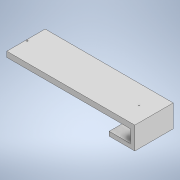
# Autodesk Inventor part: kamera_feste
Saved by Autodesk Inventor 2022 (Build 260153000, 153)
## iProperties
Created: 2022-02-27
Part Number: kamera_feste
Material: Generic
Document SubType Name: Modeling
Designer: eivin
Density: 1 g/cm^3
Appearance: Default
Author: eivin
Autodesk Inventor part; units mm, degrees
ref_plane "YZ Plane" through (0, 0, 0) normal (1, 0, 0) x (0, 1, 0)
ref_plane "XZ Plane" through (0, 0, 0) normal (0, 1, 0) x (-1, 0, 0)
ref_plane "XY Plane" through (0, 0, 0) normal (0, 0, 1) x (1, 0, 0)
sketch "Sketch1" plane through (0, 0, 0) normal (0, 0, 1) x (1, 0, 0)
  line L0 (25, -5) -> (-25, -5)
  line L1 (-25, -5) -> (-25, 5)
  line L2 (-25, 5) -> (25, 5)
  line L3 (25, -5) -> (-25, 5) construction
  line L4 (-25, -5) -> (25, 5) construction
  line L5 (25, -5) -> (35, -5)
  line L6 (35, -5) -> (35, 35)
  line L7 (25, 35) -> (25, 5)
  line L8 (25, 35) -> (-265, 35)
  line L9 (-265, 35) -> (-265, 50)
  line L10 (-265, 50) -> (35, 50)
  line L11 (35, 50) -> (35, 35)
  point P0 (0, 0)
  dimension "d0" = 50
  dimension "d1" = 10
  dimension "d2" = 10
  dimension "d3" = 40
  dimension "d4" = 300
  dimension "d5" = 15
  constraints: 24 end point, 4 parallel, 3 horizontal, 3 perpendicular, 2 midpoint
  measures "d0" distance of L2.end L1.end
  measures "d1" distance of L0.end L1.end
  measures "d2" distance of L7.start L6.end
  measures "d3" distance of L6.end L5.end
  measures "d4" distance of L9.end L10.end
  measures "d5" distance of L8.end L9.end
extrude "Extrusion1" add sketch "Sketch1" along normal mid plane 90
sketch "Sketch4" plane through (-25, -5, 45) normal (0, -1, 0) x (1, 0, 0)
  circle A0 centre (25, -45) radius 1
  dimension "d17" = 2
  constraints: 1 centre point, 1 coincident
  measures "d17" diameter of A0
extrude "Extrusion4" cut sketch "Sketch4" against normal through all
sketch "Sketch5" plane through (-265, 35, 45) normal (-1, 0, 0) x (0, 0, 1)
  line L0 (-7.5, 7) -> (-82.5, 7)
  line L1 (-82.5, 7) -> (-82.5, 2)
  line L2 (-7.5, 2) -> (-7.5, 7)
  line L3 (-7.5, 7) -> (-82.5, 2) construction
  line L4 (-82.5, 7) -> (-7.5, 2) construction
  line L5 (-72.5, 2) -> (-72.5, 0)
  line L6 (-72.5, 0) -> (-17.5, 0)
  line L7 (-17.5, 0) -> (-17.5, 2)
  line L8 (-82.5, 2) -> (-72.5, 2)
  line L9 (-17.5, 2) -> (-7.5, 2)
  point P0 (-45, -35)
  point P1 (-45, 4.5)
  dimension "d32" = 75
  dimension "d33" = 5
  dimension "d34" = 55
  constraints: 20 end point, 4 parallel, 2 midpoint, 1 horizontal, 1 perpendicular
  measures "d32" distance of L2.start L1.end
  measures "d33" distance of L1.end L0.end
  measures "d34" distance of L6.end L5.end
sketch "Sketch6" plane through (-265, 35, 45) normal (-1, 0, 0) x (0, 0, 1)
  line L0 (-90, 15) -> (0, 15) projected
  line L1 (0, 15) -> (-90, 15)
  line L2 (-90, 15) -> (-90, 12.5)
  line L3 (-90, 12.5) -> (0, 12.5)
  line L4 (0, 12.5) -> (0, 15)
  point P0 (-45, -35)
  dimension "d25" = 90
  dimension "d26" = 2.5
  constraints: 8 end point, 2 parallel, 1 horizontal, 1 perpendicular
  measures "d25" distance of L3.end L2.end
  measures "d26" distance of L2.end L1.end
extrude "Extrusion6" cut sketch "Sketch6" against normal blind 300
sketch "Sketch7" plane through (-265, 47.5, 45) normal (0, 1, 0) x (1, 0, 0)
  circle A0 centre (3, 45) radius 1.5
  point P0 (265, 45)
  dimension "d29" = 3
  constraints: 1 centre point
  measures "d29" diameter of A0
extrude "Extrusion7" cut sketch "Sketch7" against normal blind 60
extrude "Extrusion8" cut sketch "Sketch5" against normal blind 250
body "Solid1"
